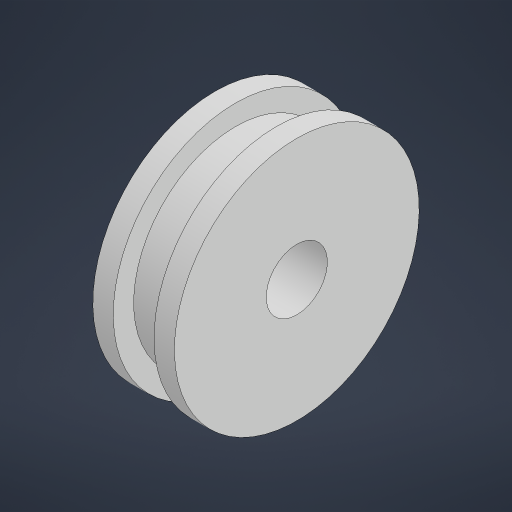
# Autodesk Inventor part: Pulley_L
Saved by Autodesk Inventor 2024.2 (Build 282272000, 272)
## iProperties
Created: 2024-02-26
Part Number: Pulley_L
Material: 一般
Document SubType Name: Modeling
Designer: Hanaoka
Density: 1 g/cm^3
Appearance: 既定
Author: Hanaoka
Autodesk Inventor part; units mm, degrees
ref_plane "YZ Plane" through (0, 0, 0) normal (1, 0, 0) x (0, 1, 0)
ref_plane "XZ Plane" through (0, 0, 0) normal (0, 1, 0) x (-1, 0, 0)
ref_plane "XY Plane" through (0, 0, 0) normal (0, 0, 1) x (1, 0, 0)
sketch "スケッチ1" plane through (0, 0, 0) normal (0, 0, 1) x (1, 0, 0)
  line L0 (-2, 6) -> (-1, 6)
  line L1 (-1, 6) -> (-1, 5)
  line L2 (-1, 5) -> (1, 5)
  line L3 (1, 5) -> (1, 6)
  line L4 (1, 6) -> (2, 6)
  line L5 (2, 6) -> (2, 1.5)
  line L6 (2, 1.5) -> (-2, 1.5)
  line L7 (-2, 1.5) -> (-2, 6)
  line L8 (0, -1.2) -> (0, 7.2) construction
  line L9 (-2.8, 0) -> (2.8, 0) projected
  point P0 (0, 0)
  dimension "d0" = 1.5
  dimension "d1" = 5
  dimension "d2" = 1
  dimension "d3" = 2
  dimension "d4" = 1
  constraints: 16 end point, 5 perpendicular, 2 point on line, 1 collinear, 1 horizontal, 1 vertical, 1 other
  measures "d0" distance from line of point (0, 0) L6
  measures "d1" distance from line of point (0, 0) L2
  measures "d2" distance of L2.end L3.end
  measures "d3" distance of L1.end L2.end
  measures "d4" distance of L3.end L4.end
revolve "回転1" add sketch "スケッチ1" angle 360 about axis through (-10, 0, 0) along (1, 0, 0)
